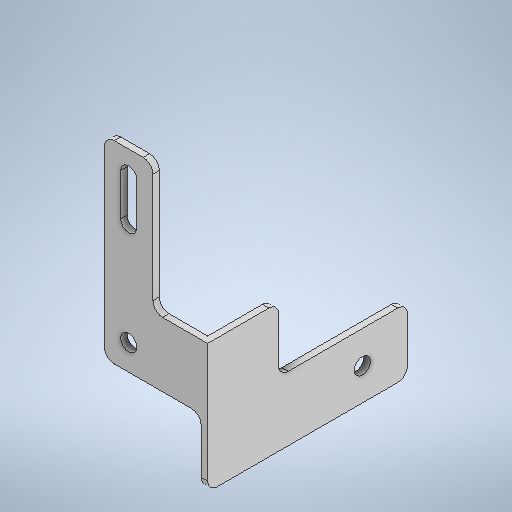
# Autodesk Inventor part: Rectangle_plate[1]
Saved by Autodesk Inventor 2025.2 (Build 292293000, 293)
## iProperties
Created: 2025-02-15
Part Number: Rectangle_plate[1]
Material: Generic
Document SubType Name: Modeling
Designer: shiva
Density: 1 g/cm^3
Appearance: Default
Author: shiva
Autodesk Inventor part; units mm, degrees
ref_plane "YZ Plane" through (0, 0, 0) normal (1, 0, 0) x (0, 1, 0)
ref_plane "XZ Plane" through (0, 0, 0) normal (0, 1, 0) x (-1, 0, 0)
ref_plane "XY Plane" through (0, 0, 0) normal (0, 0, 1) x (1, 0, 0)
sketch "Sketch1" plane through (0, 0, 0) normal (0, 0, 1) x (1, 0, 0)
  line L0 (7.5, -28.5) -> (-7.5, -28.5)
  line L1 (-7.5, -28.5) -> (-7.5, 28.5)
  line L2 (-7.5, 28.5) -> (7.5, -28.5) construction
  line L3 (7.5, 28.5) -> (-7.5, -28.5) construction
  circle A0 centre (0, -20.5) radius 2.5
  line L4 (0, 24.5) -> (0, 11.5) construction
  line L5 (-2.5, 24.5) -> (-2.5, 11.5)
  line L6 (2.5, 11.5) -> (2.5, 24.5)
  arc A1 (2.5, 24.5) -> (-2.5, 24.5) centre (0, 24.5) ccw
  arc A2 (-2.5, 11.5) -> (2.5, 11.5) centre (0, 11.5) ccw
  line L7 (7.5, 31.5) -> (-7.5, 31.5)
  line L8 (-7.5, 31.5) -> (-7.5, -28.5)
  line L9 (7.5, 31.5) -> (7.5, -28.5)
  line L10 (7.5, -8.5) -> (7.5, -28.5)
  line L11 (7.5, -28.5) -> (22.5, -28.5)
  line L12 (22.5, -28.5) -> (22.5, -8.5)
  line L13 (22.5, -8.5) -> (7.5, -8.5)
  line L14 (7.5, -8.5) -> (7.5, -28.5)
  line L15 (22.5, -28.5) -> (24.5, -28.5)
  line L16 (24.5, -28.5) -> (24.5, -8.5)
  line L17 (24.5, -8.5) -> (22.5, -8.5)
  line L18 (22.5, -8.5) -> (22.5, -28.5)
  point P0 (0, 0)
  point P1 (0, 18)
  dimension "d7" = 15
  dimension "d8" = 57
  dimension "d9" = 5
  dimension "d10" = 13
  dimension "d11" = 5
  dimension "d12" = 60
  dimension "d39" = 15
  dimension "d40" = 20
  dimension "d41" = 2
  constraints: 40 end point, 5 parallel, 4 point on circle, 4 tangent, 3 centre point, 3 midpoint, 2 horizontal, 2 perpendicular, 2 vertical, 1 collinear
  measures "d7" distance of L0.start L0.end
  measures "d8" distance of L3.start L0.start
  measures "d9" diameter of A0
  measures "d10" distance of L4.start L4.end
  measures "d11" diameter of A2
  measures "d12" distance of L0.start L7.start
  measures "d39" distance of L13.end L12.end
  measures "d40" distance of L12.end L11.end
  measures "d41" distance of L17.end L16.end
extrude "Extrusion1" add sketch "Sketch1" along normal blind 2 contours L0 L1 L8 L7 L9
extrude "Extrusion2" add sketch "Sketch1" along normal blind 2 contours L9 L13 L12 L11 | L12 L17 L16 L15
extrude "Extrusion8" add sketch "Sketch1" against normal blind 60 contours L12 L17 L16 L15
sketch "Sketch6" plane through (-7.5, -28.5, 0) normal (0, -1, 0) x (1, 0, 0)
  line L0 (32, -60) -> (32, 2) projected
  line L1 (30, 0) -> (30, -60) projected
  line L2 (32, 2) -> (30, 2)
  line L3 (30, 2) -> (30, -60)
  line L4 (30, -60) -> (32, -60)
  line L5 (32, -60) -> (32, 2)
  line L6 (30, -60) -> (32, -60)
  line L7 (32, -60) -> (32, -20)
  line L8 (32, -20) -> (30, -20)
  line L9 (30, -20) -> (30, -60)
  point P0 (7.5, 0)
  dimension "d51" = 40
  constraints: 16 end point, 4 parallel, 2 horizontal, 2 perpendicular, 1 point on line
  measures "d51" distance of L7.end L6.end
extrude "Extrusion9" cut sketch "Sketch6" against normal blind 20 contours L4 L1 L8 L0
extrude "Extrusion11" add sketch "Sketch6" along normal blind 20
sketch "Sketch8" plane through (24.5, -8.5, 2) normal (1, 0, 0) x (0, 0, -1)
  circle A0 centre (48, -30) radius 2.5
  point P0 (2, 8.5)
  dimension "d54" = 5
  constraints: 1 centre point
  measures "d54" diameter of A0
extrude "Extrusion12" cut sketch "Sketch8" against normal up to surface (2 mm away)
fillet "Fillet1" radius 3 10 edges at (23.5, -48.5, 2) (23.5, -8.5, -20) (23.5, -28.5, -20) (23.5, -28.5, -60) (23.5, -48.5, -60) (7.5, -8.5, 1) (22.5, -28.5, 1) (-7.5, -28.5, 1) (7.5, 31.5, 1) (-7.5, 31.5, 1)
body "Solid1"
